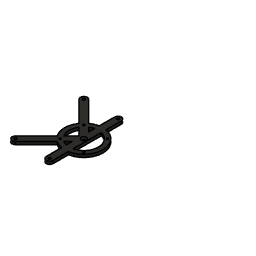
sensors-plate_lidar2d_slamtec-rplidar-s2_support (Autodesk Fusion 360 design; units mm, degrees)
Autodesk Fusion 360 part; units mm, degrees
note: some values were not read from the file. Set by a fixed rule: which sketch regions a step uses.
sketch "Sketch1" plane through (0, 392, 0) normal (0, 1, 0) x (-1, 0, 0)
  circle A0 centre (120, -60) radius 2
  circle A1 centre (0, 120) radius 2
  circle A2 centre (120, 120) radius 2
  circle A3 centre (-120, 0) radius 2
  circle A4 centre (0, -120) radius 2
  circle A5 centre (0, -60) radius 2
  circle A6 centre (165.5, 26.5835) radius 2.5
  circle A7 centre (0, 0) radius 2
  circle A8 centre (60, 120) radius 2
  circle A9 centre (-165.5, -26.5835) radius 2.5
  circle A10 centre (165.5, 78.1855) radius 2.5
  circle A11 centre (120, 0) radius 2
  circle A12 centre (120, -120) radius 2
  circle A13 centre (-60, 60) radius 2
  circle A14 centre (-60, 120) radius 2
  circle A15 centre (-120, -60) radius 2
  circle A16 centre (60, 60) radius 2
  circle A17 centre (0, 60) radius 2
  circle A18 centre (165.5, -26.5835) radius 2.5
  circle A19 centre (60, -60) radius 2
  circle A20 centre (-165.5, 26.5835) radius 2.5
  circle A21 centre (60, 0) radius 2
  circle A22 centre (120, 60) radius 2
  circle A23 centre (165.5, -78.1855) radius 2.5
  circle A24 centre (-120, 60) radius 2
  circle A25 centre (-120, 120) radius 2
  circle A26 centre (-60, -120) radius 2
  circle A27 centre (-165.5, 78.1855) radius 2.5
  circle A28 centre (-120, -120) radius 2
  circle A29 centre (-60, 0) radius 2
  circle A30 centre (60, -120) radius 2
  circle A31 centre (-165.5, -78.1855) radius 2.5
  circle A32 centre (-60, -60) radius 2
  line L0 (-176, 131) -> (-176, -131)
  line L1 (-176, -131) -> (176, -131)
  line L2 (176, -131) -> (176, 131)
  line L3 (176, 131) -> (-176, 131)
  circle A33 centre (-120, 60) radius 6
  circle A34 centre (-120, 0) radius 6
  circle A35 centre (-120, -60) radius 6
  circle A36 centre (-60, 60) radius 6
  circle A37 centre (-60, -60) radius 6
  line L4 (-126, 60) -> (-126, -60)
  line L5 (-114, -60) -> (-114, 60)
  line L6 (-64.2426, 64.2426) -> (-124.2426, 4.2426)
  line L7 (-55.7574, 55.7574) -> (-115.7574, -4.2426)
  line L8 (-64.2426, -64.2426) -> (-124.2426, -4.2426)
  line L9 (-55.7574, -55.7574) -> (-115.7574, 4.2426)
  circle A38 centre (-120, 60) radius 2.15
  circle A39 centre (-120, 0) radius 2.15
  circle A40 centre (-120, -60) radius 2.15
  circle A41 centre (-60, -60) radius 2.15
  circle A42 centre (-60, 60) radius 2.15
  circle A43 centre (-120, 0) radius 29.5 construction
  line L10 (-140.8597, 20.8597) -> (-99.1403, 20.8597) construction
  line L11 (-99.1403, 20.8597) -> (-99.1403, -20.8597) construction
  line L12 (-99.1403, -20.8597) -> (-140.8597, -20.8597) construction
  line L13 (-140.8597, -20.8597) -> (-140.8597, 20.8597) construction
  line L14 (-140.8597, 20.8597) -> (-99.1403, -20.8597) construction
  line L15 (-99.1403, 20.8597) -> (-140.8597, -20.8597) construction
  circle A44 centre (-140.8597, 20.8597) radius 1.65
  circle A45 centre (-140.8597, -20.8597) radius 1.65
  circle A46 centre (-99.1403, -20.8597) radius 1.65
  circle A47 centre (-99.1403, 20.8597) radius 1.65
  circle A48 centre (-120, 0) radius 33.5
  circle A49 centre (-120, 0) radius 25.5
  point P0 (-120, 0)
  dimension "d172" = 12
  dimension "d173" = 0.15
  dimension "d174" = 0.15
  dimension "d175" = 0.15
  dimension "d176" = 0.15
  dimension "d177" = 0.15
  dimension "d178" = 59
  dimension "d179" = 3.3
  dimension "d180" = 4
  dimension "d181" = -4
  constraint concentric A24 A33
  constraint concentric A3 A34
  constraint concentric A15 A35
  constraint concentric A13 A36
  constraint concentric A32 A37
  constraint equal A33 A36
  constraint equal A33 A34
  constraint equal A33 A35
  constraint equal A33 A37
  constraint coincident A33 L4.start
  constraint coincident A35 L4.end
  constraint coincident A35 L5.start
  constraint coincident A33 L5.end
  constraint coincident A36 L6.start
  constraint coincident A34 L6.end
  constraint coincident A36 L7.start
  constraint coincident A34 L7.end
  constraint coincident A37 L8.start
  constraint coincident A34 L8.end
  constraint coincident A37 L9.start
  constraint coincident A34 L9.end
  constraint tangent A37 L8
  constraint tangent A34 L8
  constraint tangent A34 L9
  constraint tangent A37 L9
  constraint tangent A35 L5
  constraint tangent A33 L5
  constraint tangent A33 L4
  constraint tangent A35 L4
  constraint tangent A34 L6
  constraint tangent A34 L7
  constraint tangent A36 L6
  constraint tangent A36 L7
  constraint concentric A34 A43
  constraint horizontal L10
  constraint perpendicular L10 L11
  constraint parallel L10 L12
  constraint parallel L11 L13
  constraint coincident L14 P0
  constraint coincident L15 P0
  constraint coincident A43 L10.start
  constraint coincident P0 A3.centre
  constraint equal L10 L11
  constraint coincident L10.start L13.end
  constraint coincident L12.end L13.start
  constraint coincident L11.end L12.start
  constraint coincident L10.end L11.start
  constraint equal A44 A47
  constraint equal A44 A45
  constraint equal A44 A46
  measures "d172" diameter of A33
  measures "d178" diameter of A43
  measures "d179" diameter of A44
extrude "Extrude1" add sketch "Sketch1" along normal blind 5 contours A33 | A33 L4 L5 A48 | L5 L6 A48 A49 | L4 L5 A48 A49 | L4 A48 A49 | A34 L4 L5 L6 A49 | L6 L7 A48 A49 | A36 L6 L7 A48 | A35 L4 L5 A48 | L4 L5 A48 A49 | L5 L6 L7 L9 A49 | A34 L5 L6 L9 | A36 | L7 L9 A48 A49 | A34 | A34 L4 L5 L8 A49 | A35 | L5 L8 A48 A49 | L5 L7 L9 | A34 L5 L9 | A34 L5 L7 L8 | A37 L8 L9 A48 | L8 L9 A48 A49 | A34 L5 L7 | L5 L7 L8 L9 A49 | A37
hole "Hole1" at (140.8597, 392, 20.8597) direction (0, 1, 0) diameter 3 depth 5 tip angle 180 countersink diameter 6 countersink angle 90
hole "Hole2" at (140.8597, 392, -20.8597) direction (0, 1, 0) diameter 3 depth 5 tip angle 180 countersink diameter 6 countersink angle 90
hole "Hole3" at (99.1403, 392, -20.8597) direction (0, 1, 0) diameter 3 depth 5 tip angle 180 countersink diameter 6 countersink angle 90
hole "Hole4" at (99.1403, 392, 20.8597) direction (0, 1, 0) diameter 3 depth 5 tip angle 180 countersink diameter 6 countersink angle 90
hole "Hole5" at (120, 397, 0) direction (0, -1, 0) diameter 4 depth 5 tip angle 180 countersink diameter 9 countersink angle 90
